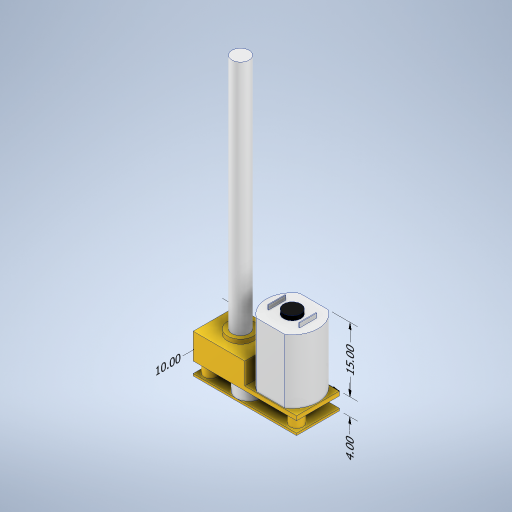
# Autodesk Inventor part: motor_M4_55
Saved by Autodesk Inventor 2024.1 (Build 281209000, 209)
## iProperties
Created: 2025-01-23
Part Number: motor_M4_55
Material: アルミニウム 6061
Document SubType Name: Modeling
Designer: hibik
Density: 2.7 g/cm^3
Appearance: アルミニウム - フラット
Author: hibik
Autodesk Inventor part; units mm, degrees
ref_plane "YZ Plane" through (0, 0, 0) normal (1, 0, 0) x (0, 1, 0)
ref_plane "XZ Plane" through (0, 0, 0) normal (0, 1, 0) x (-1, 0, 0)
ref_plane "XY Plane" through (0, 0, 0) normal (0, 0, 1) x (1, 0, 0)
sketch "スケッチ2" plane through (0, 0, 0) normal (0, 1, 0) x (-1, 0, 0)
  circle A0 centre (0, 0) radius 2
  line L0 (-6, 5) -> (6, 5)
  line L1 (6, 5) -> (6, -5)
  line L2 (6, -5) -> (-6, -5)
  line L3 (-6, -5) -> (-6, 5)
  line L4 (-6, 5) -> (6, -5) construction
  line L5 (6, 5) -> (-6, -5) construction
  line L6 (-18, 5) -> (-6, 5)
  line L7 (-6, 5) -> (-6, -5)
  line L8 (-6, -5) -> (-18, -5)
  line L9 (-18, -5) -> (-18, 5)
  line L10 (-18, 5) -> (-6, -5) construction
  line L11 (-6, 5) -> (-18, -5) construction
  point P0 (-12, 0)
  dimension "d0" = 4
  dimension "d1" = 12
  dimension "d2" = 10
  dimension "d3" = 12
  constraints: 24 end point, 4 midpoint, 4 parallel, 3 collinear, 2 horizontal, 2 perpendicular, 1 centre point, 1 coincident
  measures "d0" diameter of A0
  measures "d1" distance of L1.end L2.end
  measures "d2" distance of L0.end L1.end
  measures "d3" distance of L7.end L8.end
extrude "押し出し1" add sketch "スケッチ2" along normal blind 4 contours A0 | L0 L1 L2 L3 | L3 L8 L9 L6
extrude "押し出し2" add sketch "スケッチ2" along normal blind 9 contours A0 | L0 L1 L2 L3
extrude "押し出し3" add sketch "スケッチ2" along normal blind 65 contours A0
sketch "スケッチ3" plane through (0, 9, 0) normal (0, 1, 0) x (1, 0, 0)
  circle A0 centre (0, 0) radius 2 projected
  circle A1 centre (0, 0) radius 3
  dimension "d10" = 6
  constraints: 1 centre point, 1 coincident
  measures "d10" diameter of A1
extrude "押し出し4" add sketch "スケッチ3" along normal blind 1 contours A0 | A1
sketch "スケッチ4" plane through (0, 4, 0) normal (0, 1, 0) x (1, 0, 0)
  circle A0 centre (12, 0) radius 6
  line L0 (18, -5) -> (18, 5) projected
  line L1 (6, -5) -> (6, 5) projected
  line L2 (6, 5) -> (6, -5) projected
  line L3 (6, -5) -> (18, -5) projected
  line L4 (18, -5) -> (18, 5) projected
  line L5 (18, 5) -> (6, 5) projected
  point P0 (0, 0)
  point P1 (15.3166, 5)
  point P2 (8.6834, 5)
  point P3 (8.6834, -5)
  point P4 (15.3166, -5)
  constraints: 2 tangent, 1 centre point, 1 horizontal alignment
extrude "押し出し5" add sketch "スケッチ4" along normal blind 15 contours A0 L3 L5
sketch "スケッチ5" plane through (0, 19, 0) normal (0, 1, 0) x (1, 0, 0)
  arc A0 (8.6834, 5) -> (8.6834, -5) centre (12, 0) ccw projected
  circle A1 centre (12, 0) radius 2
  line L0 (8.3, 2) -> (8.5, 2)
  line L1 (8.5, 2) -> (8.5, -2)
  line L2 (8.5, -2) -> (8.3, -2)
  line L3 (8.3, -2) -> (8.3, 2)
  line L4 (15.5, 2) -> (15.7, 2)
  line L5 (15.7, 2) -> (15.7, -2)
  line L6 (15.7, -2) -> (15.5, -2)
  line L7 (15.5, -2) -> (15.5, 2)
  line L8 (15.3166, 5) -> (8.6834, 5) projected
  line L9 (12, 5) -> (12, 0)
  line L10 (-6, -5) -> (18, -5) projected
  point P0 (0, 0)
  point P1 (8.5, 0)
  point P2 (15.5, 0)
  dimension "d15" = 4
  dimension "d16" = 0.2
  dimension "d17" = 3.5
  constraints: 18 end point, 4 parallel, 3 midpoint, 3 perpendicular, 2 horizontal, 2 point on line, 1 centre point, 1 coincident, 1 collinear, 1 horizontal alignment, 1 other
  measures "d15" diameter of A1
  measures "d16" distance between parallel lines of L5 L7
  measures "d17" distance from line of A0.centre L1
extrude "押し出し6" add sketch "スケッチ5" along normal blind 1
sketch "スケッチ6" plane through (0, 4, 0) normal (0, 1, 0) x (1, 0, 0)
  line L0 (15.5, -2) -> (15.5, 2) projected
  line L1 (15.5, 2) -> (15.7, 2) projected
  line L2 (15.7, 2) -> (15.7, -2) projected
  line L3 (15.7, -2) -> (15.5, -2) projected
  line L4 (8.3, -2) -> (8.3, 2) projected
  line L5 (8.3, 2) -> (8.5, 2) projected
  line L6 (8.5, 2) -> (8.5, -2) projected
  line L7 (8.5, -2) -> (8.3, -2) projected
  circle A0 centre (12, 0) radius 2 projected
  arc A1 (8.6834, 5) -> (8.6834, -5) centre (12, 0) ccw projected
  line L8 (8.6834, -5) -> (15.3166, -5) projected
  arc A2 (15.3166, -5) -> (15.3166, 5) centre (12, 0) ccw projected
  line L9 (15.3166, 5) -> (8.6834, 5) projected
  circle A3 centre (12, 0) radius 5.5
  line L10 (15.1623, -4.5) -> (8.8377, -4.5)
  line L11 (8.8377, -4.5) -> (8.8377, 4.5)
  line L12 (8.8377, 4.5) -> (15.1623, 4.5)
  line L13 (15.1623, 4.5) -> (15.1623, -4.5)
  line L14 (15.1623, -4.5) -> (8.8377, 4.5) construction
  line L15 (8.8377, -4.5) -> (15.1623, 4.5) construction
  point P0 (0, 0)
  dimension "d20" = 11
  dimension "d21" = 9
  constraints: 12 end point, 2 midpoint, 2 parallel, 1 coincident, 1 horizontal, 1 perpendicular, 3 other
  measures "d21" distance of L10.end L11.end
extrude "押し出し7" cut sketch "スケッチ6" along normal blind 0.2 contours L9 A3 L8 A1 | L9 A3 L12 | A3 L10 L8 | L9 A2 L8 A3
sketch "スケッチ7" plane through (0, 0, 0) normal (0, -1, 0) x (1, 0, 0)
  line L0 (17.5, -4.5) -> (-5.5, -4.5)
  line L1 (-5.5, -4.5) -> (-5.5, 4.5)
  line L2 (-5.5, 4.5) -> (17.5, 4.5)
  line L3 (17.5, 4.5) -> (17.5, -4.5)
  line L4 (6, -5) -> (6, 5) projected
  line L5 (17.5, -4.5) -> (-5.5, 4.5) construction
  line L6 (-5.5, -4.5) -> (17.5, 4.5) construction
  line L7 (-6, -5) -> (-6, 5) projected
  line L8 (18, -5) -> (-6, -5) projected
  circle A0 centre (8, -3) radius 1.5
  circle A1 centre (16, 3) radius 1.5
  circle A2 centre (4, -3) radius 1.5
  circle A3 centre (-4, 3) radius 1.5
  line L9 (5.5, 4.5) -> (6.5, 4.5)
  line L10 (6.5, 4.5) -> (6.5, -4.5)
  line L11 (6.5, -4.5) -> (5.5, -4.5)
  line L12 (5.5, -4.5) -> (5.5, 4.5)
  line L13 (5.5, 4.5) -> (6.5, -4.5) construction
  line L14 (6.5, 4.5) -> (5.5, -4.5) construction
  line L15 (18, -5) -> (-6, -5) projected
  line L16 (18, 5) -> (18, -5) projected
  line L17 (-6, 5) -> (18, 5) projected
  line L18 (-6, -5) -> (-6, 5) projected
  point P0 (0, 0)
  point P1 (6, 0)
  dimension "d24" = 23
  dimension "d25" = 0.5
  dimension "d26" = 0.5
  dimension "d27" = 3
  dimension "d31" = 1
  constraints: 24 end point, 8 tangent, 5 midpoint, 4 centre point, 4 parallel, 3 equal radius, 2 horizontal, 2 perpendicular, 1 collinear
  measures "d24" distance of L1.end L2.end
  measures "d25" distance between parallel lines of L7 L1
  measures "d26" distance between parallel lines of L8 L0
  measures "d27" diameter of A0
  measures "d31" distance of L10.end L11.end
extrude "押し出し8" cut sketch "スケッチ7" against normal blind 3 contours L3 L2 L4 L17 L16 L8 L0 | L0 A0 L10 L2 A1 L3 | L0 L10 A0 | A1 L2 L3 | L0 L4 L2 L10 | L4 L8 L7 L17 L2 L1 L0 | L0 L12 L2 L4 | L0 A2 L12 | L0 L1 A3 L2 L12 A2 | A3 L1 L2
extrude "押し出し9" add sketch "スケッチ2" along normal blind 0.5 contours A0 | L0 L1 L2 L3 | L3 L8 L9 L6
sketch "スケッチ9" plane through (0, 0, 0) normal (0, -1, 0) x (1, 0, 0)
  circle A0 centre (4, -3) radius 1.5 projected
  circle A1 centre (4, -3) radius 1.5 projected
  circle A2 centre (4, 2) radius 3
  line L0 (-6, 5) -> (18, 5) projected
  point P0 (0, 0)
  dimension "d38" = 6
  constraints: 1 centre point, 1 tangent, 1 vertical alignment
  measures "d38" diameter of A2
extrude "押し出し10" add sketch "スケッチ9" against normal up to surface (3 mm away) contours A2
equation "\"d26\" = d25"
